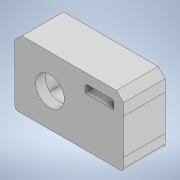
# Autodesk Inventor part: linear bearing shroud
Saved by Autodesk Inventor 2020 (Build 240168000, 168)
## iProperties
Created: 2021-02-24
Part Number: linear bearing shroud
Material: Generic
Document SubType Name: Modeling
Designer: AOB
Density: 1 g/cm^3
Appearance: Default
Mass: 4.91545 g
Surface Area: 37.8404 cm^2
Volume: 4.91545 cm^3
Author: AOB
Autodesk Inventor part; units mm, degrees
ref_plane "YZ Plane" through (0, 0, 0) normal (1, 0, 0) x (0, 1, 0)
ref_plane "XZ Plane" through (0, 0, 0) normal (0, 1, 0) x (-1, 0, 0)
sketch "Sketch1" plane through (0, 0, 0) normal (0, 0, 1) x (1, 0, 0)
  circle A0 centre (0, 0) radius 7.5
  circle A1 centre (0, 0) radius 11 construction
  line L0 (19.9999, 7) -> (19.9999, 5)
  line L1 (19.9999, 5) -> (11, 5)
  line L2 (11, 5) -> (11, 7.05)
  circle A2 centre (0, 0) radius 6.25 construction
  line L3 (19.9999, 6.25) -> (19.9999, 7) construction
  line L4 (0, 7.05) -> (0, 6.25) construction
  line L5 (11, 7) -> (11, 6.65)
  line L6 (19.4426, 7.5574) -> (11.5574, 7.5574)
  line L7 (-0.0187, 7.5) -> (-0.0187, 12.5) construction
  line L8 (-9.9738, -10.483) -> (22.0304, -10.4031)
  line L9 (23.0279, -6.4861) -> (23, 4.6722)
  line L10 (11, 7) -> (11.5574, 7.5574)
  line L11 (19.4426, 7.5574) -> (19.9999, 7)
  line L12 (-11, 8.3388) -> (-11, 0)
  line L13 (-11, 0) -> (-10.9763, -9.4855)
  line L14 (15.1283, 7.5574) -> (15.1283, 10.5574) construction
  line L15 (19.9999, 7) -> (22.9999, 7) construction
  line L16 (23.0279, -6.4861) -> (23.0279, -9.4031)
  line L17 (-8.782, 10.5568) -> (20.782, 10.5568)
  line L18 (23, 8.3389) -> (23, 4.6722)
  line L19 (-9.5, 0.0037) -> (-11, 0) construction
  line L20 (20.782, 10.5568) -> (21.8909, 9.4479) construction
  line L21 (20.782, 10.5568) -> (23, 8.3389)
  line L22 (-8.782, 10.5568) -> (-11, 8.3388)
  arc A3 (22.0304, -10.4031) -> (23.0279, -9.4031) centre (22.0279, -9.4031) ccw
  arc A4 (-10.9763, -9.4855) -> (-9.9738, -10.483) centre (-9.9763, -9.483) ccw
  line L23 (35.0262, -10.483) -> (45.0261, -10.458)
  line L24 (34, 8.3388) -> (34, 0)
  line L25 (34, 0) -> (34.0237, -9.4855)
  line L26 (36.218, 10.5568) -> (65.782, 10.5568)
  line L27 (68, 8.3389) -> (68, 7.5575)
  line L28 (65.782, 10.5568) -> (68, 8.3389)
  line L29 (36.218, 10.5568) -> (34, 8.3388)
  arc A5 (34.0237, -9.4855) -> (35.0262, -10.483) centre (35.0237, -9.483) ccw
  line L30 (68, 7.5575) -> (44.9813, 7.5)
  line L31 (45.0187, -7.5) -> (45.0261, -10.458)
  arc A6 (44.9813, 7.5) -> (45.0187, -7.5) centre (45, 0) ccw
  circle A7 centre (-48.8935, -1.0866) radius 7.5
  line L32 (-28.8936, 5.9134) -> (-28.8936, 3.9134)
  line L33 (-28.8936, 3.9134) -> (-37.8935, 3.9134)
  line L34 (-37.8935, 3.9134) -> (-37.8935, 5.9634)
  line L35 (-58.8673, -11.5696) -> (-26.8631, -11.4896)
  line L36 (-25.8656, -7.5727) -> (-25.8935, 3.5857)
  line L37 (-37.8935, 5.9134) -> (-37.336, 6.4709)
  line L38 (-29.4509, 6.4709) -> (-28.8936, 5.9134)
  line L39 (-25.8656, -7.5727) -> (-25.8656, -10.4896)
  line L40 (-25.8935, 7.2523) -> (-25.8935, 3.5857)
  arc A8 (-26.8631, -11.4896) -> (-25.8656, -10.4896) centre (-26.8656, -10.4896) ccw
  line L41 (-25.8935, 6.4709) -> (-48.9122, 6.4134)
  line L42 (-48.9122, 6.4134) -> (-48.8674, -11.5446)
  point P0 (11, 7.5574)
  point P1 (19.9999, 7.5574)
  point P2 (20, 7)
  point P3 (-11.0264, 10.5568)
  point P4 (23, 10.5568)
  point P5 (-11, 10.5568)
  point P6 (-28.8936, 5.1634)
  dimension "d1" = 22
  dimension "d5" = 12.5
  dimension "d7" = 15
  dimension "d74" = 15
  dimension "d2" = 9
  dimension "d4" = 2
  dimension "d63" = 3
  dimension "d64" = 3
  dimension "d69" = 2.218
  dimension "d71" = 1
  dimension "d72" = 9
  dimension "d73" = 2
  dimension "d75" = 1
  constraints: 86 end point, 15 point on line, 10 point on circle, 9 perpendicular, 8 tangent, 5 centre point, 5 parallel, 4 horizontal, 4 vertical, 3 coincident, 1 equal radius, 1 horizontal alignment, 1 vertical alignment, 11 other
  measures "d2" distance of L0.start L2.end
  measures "d4" distance of L0.start L0.end
  measures "d63" distance of L14.start L14.end
  measures "d64" distance of L0.start L15.end
  measures "d69" distance of L17.start point (-11, 10.557)
  measures "d71" radius of A3
  measures "d72" distance of L38.end L34.end
  measures "d73" distance of L38.end L33.start
  measures "d75" radius of A8
extrude "Extrusion1" add sketch "Sketch1" along normal blind 13 contours L0 L1 L2 L10 L6 L11 | A4 L13 L12 L22 L17 L21 L18 L9 L16 A3 L8
sketch "Sketch3" plane through (0, 0, 0) normal (0, 0, -1) x (-1, 0, 0)
  line L0 (5.7462, -7.5816) -> (-20, -7.5816)
  line L1 (-20, 7) -> (-19.4425, 7.5575)
  line L2 (9.9738, -10.483) -> (-22.0304, -10.4031) construction
  circle A0 centre (0, 0) radius 4.5
  line L3 (4.7191, 7.5575) -> (-19.4425, 7.5575)
  line L4 (-20, -7.5816) -> (-20, 7)
  line L5 (4.7191, 7.5575) -> (6.9962, 7.5575)
  line L6 (7.4962, 7.0575) -> (7.4962, -7.5816)
  line L7 (7.4962, -7.5816) -> (5.7462, -7.5816)
  line L8 (6.9962, 7.5575) -> (7.4962, 7.0575)
  point P0 (-23, -10.4856)
  point P1 (9, -10.4856)
  point P2 (-20, 5.05)
  point P3 (-23.0256, -5.5821)
  point P4 (-25, 9.0147)
  point P5 (9, 9.0147)
  point P6 (7.4962, 7.5575)
  point P7 (-22.0304, -10.4031)
  dimension "d44" = 9
  dimension "d61" = 0.5
  dimension "d62" = 0.5
  constraints: 16 end point, 3 perpendicular, 2 horizontal, 2 point on line, 1 centre point, 1 other
  measures "d44" diameter of A0
  measures "d61" distance of L5.end point (7.496, 7.557)
  measures "d62" distance of L6.start point (7.496, 7.557)
extrude "Extrusion3" cut sketch "Sketch3" against normal blind 10
extrude "Extrusion7" cut sketch "Sketch1" along normal blind 13 contours L0 L1 L2 L10 L6 L11
sketch "Sketch6" plane through (0, 0, 13) normal (0, 0, 1) x (1, 0, 0)
  circle A0 centre (0, 0) radius 4.4721
  circle A1 centre (0, 0) radius 7.5
  dimension "d78" = 8.9443
  constraints: 2 centre point, 2 coincident
  measures "d78" diameter of A0
extrude "Extrusion8" add sketch "Sketch6" against normal blind 3
ref_plane "Work Plane3" through (0, 0, 0) normal (0, 0, -1) x (-1, 0, 0)
mirror "Mirror1" about plane through (0, 0, 0) normal (0, 0, -1) of "Extrusion1", "Extrusion3", "Extrusion7", "Extrusion8"
sketch "Sketch7" plane through (20, -7.5816, 10) normal (-1, 0, 0) x (0, 0, 1)
  circle A0 centre (-10, 7.5816) radius 2.5
  dimension "d82" = 5
  constraints: 1 centre point, 1 coincident
  measures "d82" diameter of A0
extrude "Extrusion9" add sketch "Sketch7" along normal blind 12
split "Split1" plane through (0, 0, 0) removes the side toward (0, 0, -1)
equation "\"d62\" = d61"
body "Solid1"
